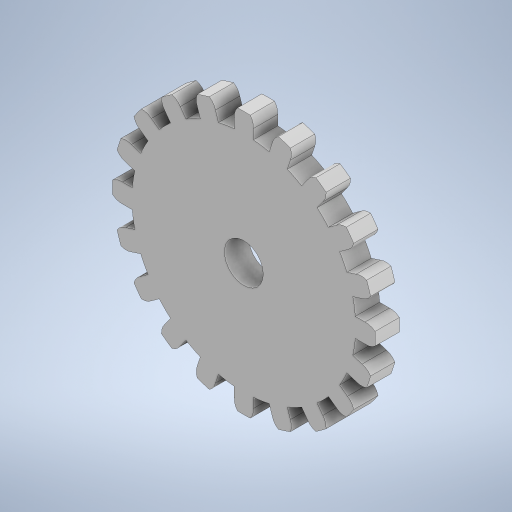
# Autodesk Inventor part: Ger
Saved by Autodesk Inventor 2024 (Build 280153000, 153)
## iProperties
Created: 2024-09-09
Part Number: Ger
Material: Generic
Document SubType Name: Modeling
Designer: srira
Density: 1 g/cm^3
Appearance: Default
Author: srira
Autodesk Inventor part; units mm, degrees
ref_plane "YZ Plane" through (0, 0, 0) normal (1, 0, 0) x (0, 1, 0)
ref_plane "XZ Plane" through (0, 0, 0) normal (0, 1, 0) x (-1, 0, 0)
ref_plane "XY Plane" through (0, 0, 0) normal (0, 0, 1) x (1, 0, 0)
sketch "Sketch1" plane through (0, 0, 0) normal (0, 0, 1) x (1, 0, 0)
  arc A0 (2.6026, 53.9372) -> (-2.6026, 53.9372) centre (0, 0) ccw
  line L0 (0, 0) -> (-3.923, 49.8459) construction
  line L1 (0, 0) -> (50, 0) construction
  line L2 (0, 0) -> (3.923, 49.8459) construction
  arc A1 (-2.6026, 53.9372) -> (-3.923, 49.8459) centre (1.5551, 50.3367) ccw
  line L3 (-3.923, 49.8459) -> (-2.3839, 54.0745) construction
  line L4 (-3.923, 49.8459) -> (0.577, 49.8459) construction
  arc A2 (3.923, 49.8459) -> (2.6026, 53.9372) centre (-1.5551, 50.3367) ccw
  line L5 (3.923, 49.8459) -> (2.3839, 54.0745) construction
  line L6 (3.923, 49.8459) -> (8.423, 49.8459) construction
  line L7 (-3.923, 49.8459) -> (-3.923, 45.8324)
  line L8 (3.923, 49.8459) -> (3.923, 45.8324)
  line L9 (-11.6723, 48.6185) -> (-10.432, 44.8015)
  arc A3 (-11.6723, 48.6185) -> (-14.1923, 52.1016) centre (-17.0339, 47.3925) ccw
  arc A4 (-14.1923, 52.1016) -> (-19.1427, 50.4931) centre (0, 0) ccw
  arc A5 (-19.1427, 50.4931) -> (-19.1342, 46.194) centre (-14.0759, 48.3536) ccw
  line L10 (0, 0) -> (-19.1342, 46.194) construction
  line L11 (-19.1342, 46.194) -> (-17.8939, 42.377)
  line L12 (-26.1249, 42.632) -> (-23.7659, 39.3851)
  arc A6 (-26.1249, 42.632) -> (-29.598, 45.1659) centre (-30.8453, 39.8092) ccw
  arc A7 (-29.598, 45.1659) -> (-33.809, 42.1064) centre (0, 0) ccw
  arc A8 (-33.809, 42.1064) -> (-32.4724, 38.0203) centre (-28.3291, 41.6373) ccw
  line L13 (0, 0) -> (-32.4724, 38.0203) construction
  line L14 (-32.4724, 38.0203) -> (-30.1134, 34.7733)
  line L15 (-38.0203, 32.4724) -> (-34.7733, 30.1134)
  arc A9 (-38.0203, 32.4724) -> (-42.1064, 33.809) centre (-41.6373, 28.3291) ccw
  arc A10 (-42.1064, 33.809) -> (-45.1659, 29.598) centre (0, 0) ccw
  arc A11 (-45.1659, 29.598) -> (-42.632, 26.1249) centre (-39.8092, 30.8453) ccw
  line L16 (0, 0) -> (-42.632, 26.1249) construction
  line L17 (-42.632, 26.1249) -> (-39.3851, 23.7659)
  line L18 (-46.194, 19.1342) -> (-42.377, 17.8939)
  arc A12 (-46.194, 19.1342) -> (-50.4931, 19.1427) centre (-48.3536, 14.0759) ccw
  arc A13 (-50.4931, 19.1427) -> (-52.1016, 14.1923) centre (0, 0) ccw
  arc A14 (-52.1016, 14.1923) -> (-48.6185, 11.6723) centre (-47.3925, 17.0339) ccw
  line L19 (0, 0) -> (-48.6185, 11.6723) construction
  line L20 (-48.6185, 11.6723) -> (-44.8015, 10.432)
  line L21 (-49.8459, 3.923) -> (-45.8324, 3.923)
  arc A15 (-49.8459, 3.923) -> (-53.9372, 2.6026) centre (-50.3367, -1.5551) ccw
  arc A16 (-53.9372, 2.6026) -> (-53.9372, -2.6026) centre (0, 0) ccw
  arc A17 (-53.9372, -2.6026) -> (-49.8459, -3.923) centre (-50.3367, 1.5551) ccw
  line L22 (0, 0) -> (-49.8459, -3.923) construction
  line L23 (-49.8459, -3.923) -> (-45.8324, -3.923)
  line L24 (-48.6185, -11.6723) -> (-44.8015, -10.432)
  arc A18 (-48.6185, -11.6723) -> (-52.1016, -14.1923) centre (-47.3925, -17.0339) ccw
  arc A19 (-52.1016, -14.1923) -> (-50.4931, -19.1427) centre (0, 0) ccw
  arc A20 (-50.4931, -19.1427) -> (-46.194, -19.1342) centre (-48.3536, -14.0759) ccw
  line L25 (0, 0) -> (-46.194, -19.1342) construction
  line L26 (-46.194, -19.1342) -> (-42.377, -17.8939)
  line L27 (-42.632, -26.1249) -> (-39.3851, -23.7659)
  arc A21 (-42.632, -26.1249) -> (-45.1659, -29.598) centre (-39.8092, -30.8453) ccw
  arc A22 (-45.1659, -29.598) -> (-42.1064, -33.809) centre (0, 0) ccw
  arc A23 (-42.1064, -33.809) -> (-38.0203, -32.4724) centre (-41.6373, -28.3291) ccw
  line L28 (0, 0) -> (-38.0203, -32.4724) construction
  line L29 (-38.0203, -32.4724) -> (-34.7733, -30.1134)
  line L30 (-32.4724, -38.0203) -> (-30.1134, -34.7733)
  arc A24 (-32.4724, -38.0203) -> (-33.809, -42.1064) centre (-28.3291, -41.6373) ccw
  arc A25 (-33.809, -42.1064) -> (-29.598, -45.1659) centre (0, 0) ccw
  arc A26 (-29.598, -45.1659) -> (-26.1249, -42.632) centre (-30.8453, -39.8092) ccw
  line L31 (0, 0) -> (-26.1249, -42.632) construction
  line L32 (-26.1249, -42.632) -> (-23.7659, -39.3851)
  line L33 (-19.1342, -46.194) -> (-17.8939, -42.377)
  arc A27 (-19.1342, -46.194) -> (-19.1427, -50.4931) centre (-14.0759, -48.3536) ccw
  arc A28 (-19.1427, -50.4931) -> (-14.1923, -52.1016) centre (0, 0) ccw
  arc A29 (-14.1923, -52.1016) -> (-11.6723, -48.6185) centre (-17.0339, -47.3925) ccw
  line L34 (0, 0) -> (-11.6723, -48.6185) construction
  line L35 (-11.6723, -48.6185) -> (-10.432, -44.8015)
  line L36 (-3.923, -49.8459) -> (-3.923, -45.8324)
  arc A30 (-3.923, -49.8459) -> (-2.6026, -53.9372) centre (1.5551, -50.3367) ccw
  arc A31 (-2.6026, -53.9372) -> (2.6026, -53.9372) centre (0, 0) ccw
  arc A32 (2.6026, -53.9372) -> (3.923, -49.8459) centre (-1.5551, -50.3367) ccw
  line L37 (0, 0) -> (3.923, -49.8459) construction
  line L38 (3.923, -49.8459) -> (3.923, -45.8324)
  line L39 (11.6723, -48.6185) -> (10.432, -44.8015)
  arc A33 (11.6723, -48.6185) -> (14.1923, -52.1016) centre (17.0339, -47.3925) ccw
  arc A34 (14.1923, -52.1016) -> (19.1427, -50.4931) centre (0, 0) ccw
  arc A35 (19.1427, -50.4931) -> (19.1342, -46.194) centre (14.0759, -48.3536) ccw
  line L40 (0, 0) -> (19.1342, -46.194) construction
  line L41 (19.1342, -46.194) -> (17.8939, -42.377)
  line L42 (26.1249, -42.632) -> (23.7659, -39.3851)
  arc A36 (26.1249, -42.632) -> (29.598, -45.1659) centre (30.8453, -39.8092) ccw
  arc A37 (29.598, -45.1659) -> (33.809, -42.1064) centre (0, 0) ccw
  arc A38 (33.809, -42.1064) -> (32.4724, -38.0203) centre (28.3291, -41.6373) ccw
  line L43 (0, 0) -> (32.4724, -38.0203) construction
  line L44 (32.4724, -38.0203) -> (30.1134, -34.7733)
  line L45 (38.0203, -32.4724) -> (34.7733, -30.1134)
  arc A39 (38.0203, -32.4724) -> (42.1064, -33.809) centre (41.6373, -28.3291) ccw
  arc A40 (42.1064, -33.809) -> (45.1659, -29.598) centre (0, 0) ccw
  arc A41 (45.1659, -29.598) -> (42.632, -26.1249) centre (39.8092, -30.8453) ccw
  line L46 (0, 0) -> (42.632, -26.1249) construction
  line L47 (42.632, -26.1249) -> (39.3851, -23.7659)
  line L48 (46.194, -19.1342) -> (42.377, -17.8939)
  arc A42 (46.194, -19.1342) -> (50.4931, -19.1427) centre (48.3536, -14.0759) ccw
  arc A43 (50.4931, -19.1427) -> (52.1016, -14.1923) centre (0, 0) ccw
  arc A44 (52.1016, -14.1923) -> (48.6185, -11.6723) centre (47.3925, -17.0339) ccw
  line L49 (0, 0) -> (48.6185, -11.6723) construction
  line L50 (48.6185, -11.6723) -> (44.8015, -10.432)
  line L51 (49.8459, -3.923) -> (45.8324, -3.923)
  arc A45 (49.8459, -3.923) -> (53.9372, -2.6026) centre (50.3367, 1.5551) ccw
  arc A46 (53.9372, -2.6026) -> (53.9372, 2.6026) centre (0, 0) ccw
  arc A47 (53.9372, 2.6026) -> (49.8459, 3.923) centre (50.3367, -1.5551) ccw
  line L52 (0, 0) -> (49.8459, 3.923) construction
  line L53 (49.8459, 3.923) -> (45.8324, 3.923)
  line L54 (48.6185, 11.6723) -> (44.8015, 10.432)
  arc A48 (48.6185, 11.6723) -> (52.1016, 14.1923) centre (47.3925, 17.0339) ccw
  arc A49 (52.1016, 14.1923) -> (50.4931, 19.1427) centre (0, 0) ccw
  arc A50 (50.4931, 19.1427) -> (46.194, 19.1342) centre (48.3536, 14.0759) ccw
  line L55 (0, 0) -> (46.194, 19.1342) construction
  line L56 (46.194, 19.1342) -> (42.377, 17.8939)
  line L57 (42.632, 26.1249) -> (39.3851, 23.7659)
  arc A51 (42.632, 26.1249) -> (45.1659, 29.598) centre (39.8092, 30.8453) ccw
  arc A52 (45.1659, 29.598) -> (42.1064, 33.809) centre (0, 0) ccw
  arc A53 (42.1064, 33.809) -> (38.0203, 32.4724) centre (41.6373, 28.3291) ccw
  line L58 (0, 0) -> (38.0203, 32.4724) construction
  line L59 (38.0203, 32.4724) -> (34.7733, 30.1134)
  line L60 (32.4724, 38.0203) -> (30.1134, 34.7733)
  arc A54 (32.4724, 38.0203) -> (33.809, 42.1064) centre (28.3291, 41.6373) ccw
  arc A55 (33.809, 42.1064) -> (29.598, 45.1659) centre (0, 0) ccw
  arc A56 (29.598, 45.1659) -> (26.1249, 42.632) centre (30.8453, 39.8092) ccw
  line L61 (0, 0) -> (26.1249, 42.632) construction
  line L62 (26.1249, 42.632) -> (23.7659, 39.3851)
  line L63 (19.1342, 46.194) -> (17.8939, 42.377)
  arc A57 (19.1342, 46.194) -> (19.1427, 50.4931) centre (14.0759, 48.3536) ccw
  arc A58 (19.1427, 50.4931) -> (14.1923, 52.1016) centre (0, 0) ccw
  arc A59 (14.1923, 52.1016) -> (11.6723, 48.6185) centre (17.0339, 47.3925) ccw
  line L64 (0, 0) -> (11.6723, 48.6185) construction
  line L65 (11.6723, 48.6185) -> (10.432, 44.8015)
  arc A60 (-3.6091, 45.8582) -> (-10.432, 44.8015) centre (0, 0) ccw
  arc A61 (10.7385, 44.729) -> (3.6091, 45.8582) centre (0, 0) ccw
  arc A62 (24.0349, 39.2214) -> (17.8939, 42.377) centre (0, 0) ccw
  arc A63 (34.9787, 29.8746) -> (30.1134, 34.7733) centre (0, 0) ccw
  arc A64 (42.4985, 17.6034) -> (39.3851, 23.7659) centre (0, 0) ccw
  arc A65 (46, 0) -> (44.8015, 10.432) centre (0, 0) ccw
  arc A66 (44.729, -10.7385) -> (45.8324, -3.923) centre (0, 0) ccw
  arc A67 (39.2214, -24.0349) -> (42.377, -17.8939) centre (0, 0) ccw
  arc A68 (29.8746, -34.9787) -> (34.7733, -30.1134) centre (0, 0) ccw
  arc A69 (17.6034, -42.4985) -> (23.7659, -39.3851) centre (0, 0) ccw
  arc A70 (3.6091, -45.8582) -> (10.432, -44.8015) centre (0, 0) ccw
  arc A71 (-10.7385, -44.729) -> (-3.923, -45.8324) centre (0, 0) ccw
  arc A72 (-24.0349, -39.2214) -> (-17.8939, -42.377) centre (0, 0) ccw
  arc A73 (-34.9787, -29.8746) -> (-30.1134, -34.7733) centre (0, 0) ccw
  arc A74 (-42.4985, -17.6034) -> (-39.3851, -23.7659) centre (0, 0) ccw
  arc A75 (-45.8582, -3.6091) -> (-44.8015, -10.432) centre (0, 0) ccw
  arc A76 (-44.729, 10.7385) -> (-45.8324, 3.923) centre (0, 0) ccw
  arc A77 (-39.2214, 24.0349) -> (-42.377, 17.8939) centre (0, 0) ccw
  arc A78 (-17.6034, 42.4985) -> (-23.7659, 39.3851) centre (0, 0) ccw
  arc A79 (-29.8746, 34.9787) -> (-34.7733, 30.1134) centre (0, 0) ccw
  arc A80 (-50, 0) -> (-49.8459, -3.923) centre (0, 0) ccw
  arc A81 (49.8459, -3.923) -> (50, 0) centre (0, 0) ccw
  point P0 (45.8582, 3.6091)
  dimension "d2" = 108
  dimension "d3" = 94.5
  dimension "d4" = 4.5
  dimension "d5" = 70
  dimension "d6" = 5.5
  dimension "d7" = 4.5
  dimension "d8" = 110
  dimension "d9" = 5.5
  dimension "d12" = 360
  constraints: 166 point on circle, 132 end point, 82 centre point, 23 point on line, 3 coincident, 3 equal length, 3 horizontal, 1 parallel, 1 perpendicular, 321 other
  measures "d2" diameter of A0
  measures "d3" angle of L1 L0
  measures "d4" distance of L0.end L3.end
  measures "d5" angle of L4 L3
  measures "d6" radius of A1
  measures "d7" distance of L2.end L5.end
  measures "d8" angle of L6 L5
  measures "d9" radius of A2
extrude "Extrusion1" add sketch "Sketch1" along normal blind 10
sketch "Sketch2" plane through (0, 0, 10) normal (0, 0, 1) x (1, 0, 0)
  circle A0 centre (0, 0) radius 8
  dimension "d16" = 16
  constraints: 1 centre point, 1 coincident
  measures "d16" diameter of A0
extrude "Extrusion2" cut sketch "Sketch2" against normal blind 10
body "Solid1"
